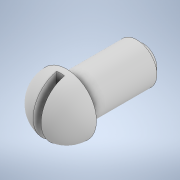
# Autodesk Inventor part: Parafuso da Valvula
Saved by Autodesk Inventor 2020 (Build 240168000, 168)
## iProperties
Created: 2022-04-26
Part Number: Parafuso da Valvula
Material: Genérico
Document SubType Name: Modeling
Designer: robofei
Density: 1 g/cm^3
Appearance: Padrão
Author: robofei
Autodesk Inventor part; units mm, degrees
ref_plane "YZ Plane" through (0, 0, 0) normal (1, 0, 0) x (0, 1, 0)
ref_plane "XZ Plane" through (0, 0, 0) normal (0, 1, 0) x (-1, 0, 0)
ref_plane "XY Plane" through (0, 0, 0) normal (0, 0, 1) x (1, 0, 0)
sketch "Esboço1" plane through (0, 0, 0) normal (0, 0, 1) x (1, 0, 0)
  circle A0 centre (0, 0) radius 10
  dimension "d0" = 20
  constraints: 1 centre point, 1 coincident
  measures "d0" diameter of A0
extrude "Extrusão1" add sketch "Esboço1" along normal blind 38
chamfer "Chanfro1" distance 3 angle 45 1 edges at (-10, 0, 0)
sketch "Esboço3" plane through (0, 0, 0) normal (0, 1, 0) x (-1, 0, 0)
  line L0 (10, 38) -> (-10, 38) projected
  arc A0 (14.87, 38) -> (-14.87, 38) centre (0, 38) ccw
  line L1 (0, 52.87) -> (0, 38)
  line L2 (-14.87, 38) -> (14.87, 38)
  point P0 (0, 0)
  dimension "d7" = 29.74
  constraints: 4 end point, 3 point on circle, 2 point on line, 1 centre point, 1 midpoint, 1 vertical
  measures "d7" diameter of A0
revolve "Revolução1" add sketch "Esboço3" angle 360 about axis through (0, 0, 52.87) along (0, 0, -1) picked at (-6.4238, 41.8753) contours L0 L2 A0 L1
sketch "Esboço4" plane through (0, 0, 0) normal (0, 1, 0) x (-1, 0, 0)
  line L0 (-2, 57) -> (2, 57)
  line L1 (2, 57) -> (2, 41)
  line L2 (2, 41) -> (-2, 41)
  line L3 (-2, 41) -> (-2, 57)
  line L4 (7, 0) -> (-7, 0) projected
  point P0 (0, 0)
  point P1 (0, 0)
  dimension "d9" = 4
  dimension "d10" = 16
  dimension "d11" = 41
  dimension "d13" = 2
  constraints: 8 end point, 2 parallel, 1 coincident, 1 horizontal, 1 perpendicular
  measures "d9" distance of L0.start L0.end
  measures "d10" distance of L0.end L1.end
  measures "d11" distance between parallel lines of L4 L2
  measures "d13" horizontal distance of L0.end point (0, 0)
extrude "Extrusão2" cut sketch "Esboço4" along normal mid plane 38
